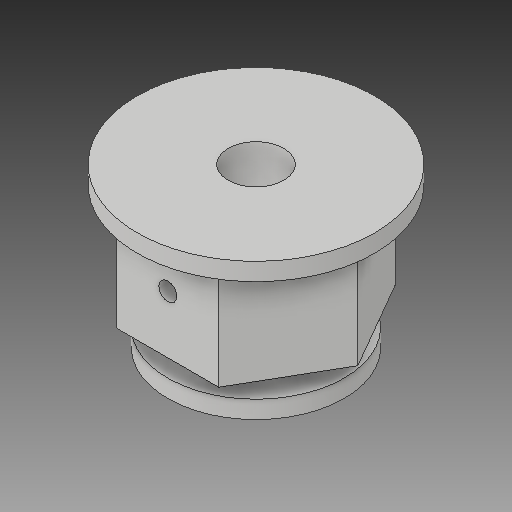
# Autodesk Inventor part: T40_hub_40mm_1screw
Saved by Autodesk Inventor 2019 (Build 230136000, 136)
## iProperties
Created: 2017-02-14
Part Number: T40_hub_40mm_1screw
Material: Générique
Document SubType Name: Modeling
Designer: Aegir
Density: 1 g/cm^3
Appearance: Par défaut
Author: Aegir
Autodesk Inventor part; units mm, degrees
ref_plane "YZ Plane" through (0, 0, 0) normal (1, 0, 0) x (0, 1, 0)
ref_plane "XZ Plane" through (0, 0, 0) normal (0, 1, 0) x (-1, 0, 0)
ref_plane "XY Plane" through (0, 0, 0) normal (0, 0, 1) x (1, 0, 0)
sketch "Esquisse1" plane through (0, 0, 0) normal (0, 1, 0) x (-1, 0, 0)
  circle A0 centre (0, 0) radius 2
  line L0 (7.3323, 0) -> (3.6662, -6.35)
  line L1 (3.6662, -6.35) -> (-3.6662, -6.35)
  line L2 (-3.6662, -6.35) -> (-7.3323, 0)
  line L3 (-7.3323, 0) -> (-3.6662, 6.35)
  line L4 (-3.6662, 6.35) -> (3.6662, 6.35)
  line L5 (3.6662, 6.35) -> (7.3323, 0)
  dimension "d0" = 12.7
  dimension "d1" = 4
  constraints: 12 end point, 2 coincident, 1 centre point, 13 other
  measures "d0" distance between parallel lines of L3 L0
  measures "d1" diameter of A0
extrude "Extrusion1" add sketch "Esquisse1" along normal blind 7.62
sketch "Esquisse2" plane through (0, 7.62, 0) normal (0, 1, 0) x (1, 0, 0)
  circle A0 centre (0, 0) radius 8.5509
  circle A1 centre (0, 0) radius 2
  constraints: 2 centre point, 2 coincident
extrude "Extrusion2" add sketch "Esquisse2" along normal blind 1.27
sketch "Esquisse3" plane through (0, 0, 0) normal (0, -1, 0) x (1, 0, 0)
  circle A0 centre (0, 0) radius 4.0595
  circle A1 centre (0, 0) radius 2
  constraints: 2 centre point, 2 coincident
extrude "Extrusion3" add sketch "Esquisse3" along normal blind 1.27
sketch "Esquisse4" plane through (0, -1.27, 0) normal (0, -1, 0) x (1, 0, 0)
  circle A0 centre (0, 0) radius 6.35
  line L0 (7.3323, 0) -> (3.6662, 6.35) projected
  circle A1 centre (0, 0) radius 2
  constraints: 2 centre point, 2 coincident, 1 tangent
extrude "Extrusion4" add sketch "Esquisse4" along normal blind 1.27
sketch "Esquisse5" plane through (-3.6662, 0, 6.35) normal (0, 0, 1) x (1, 0, 0)
  circle A0 centre (3.6662, 4.1459) radius 0.6492
  point P0 (3.6662, 0)
  constraints: 1 centre point
extrude "Extrusion5" cut sketch "Esquisse5" against normal blind 6
